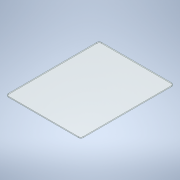
# Autodesk Inventor part: Puerta Lateral Izquierda
Saved by Autodesk Inventor 2020 (Build 240168000, 168)
## iProperties
Created: 2020-07-27
Part Number: Puerta Lateral Izquierda
Material: Genérico
Document SubType Name: Modeling
Designer: Pipi
Density: 1 g/cm^3
Appearance: Claro
Author: Pipi
Autodesk Inventor part; units mm, degrees
ref_plane "YZ Plane" through (0, 0, 0) normal (1, 0, 0) x (0, 1, 0)
ref_plane "XZ Plane" through (0, 0, 0) normal (0, 1, 0) x (-1, 0, 0)
ref_plane "XY Plane" through (0, 0, 0) normal (0, 0, 1) x (1, 0, 0)
sketch "Boceto1" plane through (0, 0, 0) normal (0, 1, 0) x (-1, 0, 0)
  line L0 (63.9389, -223.5898) -> (-164.0611, -223.5898)
  line L1 (-172.0611, -215.5898) -> (-172.0611, 72.4102)
  line L2 (-164.0611, 80.4102) -> (63.9389, 80.4102)
  line L3 (71.9389, 72.4102) -> (71.9389, -215.5898)
  arc A0 (63.9389, -223.5898) -> (71.9389, -215.5898) centre (63.9389, -215.5898) ccw
  arc A1 (-172.0611, -215.5898) -> (-164.0611, -223.5898) centre (-164.0611, -215.5898) ccw
  arc A2 (-164.0611, 80.4102) -> (-172.0611, 72.4102) centre (-164.0611, 72.4102) ccw
  arc A3 (71.9389, 72.4102) -> (63.9389, 80.4102) centre (63.9389, 72.4102) ccw
  point P0 (-172.0611, 80.4102)
  point P1 (-172.0611, -223.5898)
  point P2 (71.9389, 80.4102)
  dimension "d0" = 244
  dimension "d1" = 304
  dimension "d2" = 8
  constraints: 8 end point, 8 point on circle, 8 tangent, 6 point on line, 4 centre point, 3 equal radius, 2 parallel, 1 horizontal, 1 perpendicular
  measures "d0" distance of point (-172.061, 80.41) point (71.939, 80.41)
  measures "d1" distance of point (-172.061, -223.59) point (-172.061, 80.41)
  measures "d2" radius of A0
extrude "Extrusión1" add sketch "Boceto1" along normal blind 3
